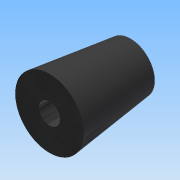
# Autodesk Inventor part: crampon
Saved by Autodesk Inventor 2015 (Build 190159000, 159)
## iProperties
Created: 2015-06-08
Part Number: crampon
Material: Générique
Document SubType Name: Modeling
Designer: Gregwar
Density: 1 g/cm^3
Appearance: Par défaut
Author: Gregwar
Autodesk Inventor part; units mm, degrees
ref_plane "YZ Plane" through (0, 0, 0) normal (1, 0, 0) x (0, 1, 0)
ref_plane "XZ Plane" through (0, 0, 0) normal (0, 1, 0) x (-1, 0, 0)
ref_plane "XY Plane" through (0, 0, 0) normal (0, 0, 1) x (1, 0, 0)
sketch "Esquisse1" plane through (0, 0, 0) normal (0, 1, 0) x (-1, 0, 0)
  circle A0 centre (0, 0) radius 6
  dimension "d0" = 12
  constraints: 1 centre point, 1 coincident
  measures "d0" diameter of A0
extrude "Extrusion1" add sketch "Esquisse1" along normal blind 20
draft "Dépouille de face1" angle 7 pull direction (0, 1, 0) faces at (-5.9223, 13.3333, -0.9625) fixed edges at (6, 20, 0)
sketch "Esquisse2" plane through (0, 20, 0) normal (0, 1, 0) x (1, 0, 0)
  circle A0 centre (0, 0) radius 6 construction
  circle A1 centre (0, 0) radius 2.6
  dimension "d4" = 5.2
  constraints: 1 centre point, 1 coincident
  measures "d4" diameter of A1
extrude "Extrusion2" cut sketch "Esquisse2" against normal through all
sketch "Esquisse3" plane through (0, 20, 0) normal (0, 1, 0) x (1, 0, 0)
  circle A0 centre (0, 0) radius 2.6 construction
  line L0 (-4, 2.3094) -> (0, 4.6188)
  line L1 (0, 4.6188) -> (4, 2.3094)
  line L2 (4, 2.3094) -> (4, -2.3094)
  line L3 (4, -2.3094) -> (0, -4.6188)
  line L4 (0, -4.6188) -> (-4, -2.3094)
  line L5 (-4, -2.3094) -> (-4, 2.3094)
  line L6 (0, 0) -> (0, 16.8814) construction
  dimension "d8" = 8
  constraints: 14 end point, 1 coincident, 1 parallel, 1 vertical, 13 other
  measures "d8" distance between parallel lines of L2 L5
extrude "Extrusion3" cut sketch "Esquisse3" against normal blind 3.5
